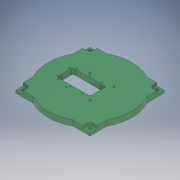
# Autodesk Inventor part: 000.202 - Крышка
Saved by Autodesk Inventor 2019 (Build 230136000, 136)
## iProperties
Created: 2020-03-17
Part Number: 000.202 - Крышка
Material: Пластик АБС
Document SubType Name: Modeling
Designer: Петров Иван
Density: 1.06 g/cm^3
Appearance: Гладкий — темный цвет морской волны
Author: Петров Иван
Autodesk Inventor part; units mm, degrees
ref_plane "YZ Plane" through (0, 0, 0) normal (1, 0, 0) x (0, 1, 0)
ref_plane "XZ Plane" through (0, 0, 0) normal (0, 1, 0) x (-1, 0, 0)
ref_plane "XY Plane" through (0, 0, 0) normal (0, 0, 1) x (1, 0, 0)
sketch "Эскиз1" plane through (0, 0, 0) normal (0, 0, 1) x (1, 0, 0)
  circle A0 centre (59.533, -59.533) radius 3 projected
  circle A1 centre (-59.533, -59.533) radius 3 projected
  circle A2 centre (-59.533, 59.533) radius 3 projected
  circle A3 centre (59.533, 59.533) radius 3 projected
  circle A4 centre (0, 0) radius 65 projected
  arc A5 (35.5618, 66.033) -> (-35.5618, 66.033) centre (0, 0) ccw projected
  line L0 (-35.5618, 66.033) -> (-66.033, 66.033) projected
  line L1 (-66.033, 66.033) -> (-66.033, 35.5618) projected
  arc A6 (-66.033, 35.5618) -> (-66.033, -35.5618) centre (0, 0) ccw projected
  line L2 (-66.033, -35.5618) -> (-66.033, -66.033) projected
  line L3 (-66.033, -66.033) -> (-35.5618, -66.033) projected
  arc A7 (-35.5618, -66.033) -> (35.5618, -66.033) centre (0, 0) ccw projected
  line L4 (35.5618, -66.033) -> (66.033, -66.033) projected
  line L5 (66.033, -66.033) -> (66.033, -35.5618) projected
  arc A8 (66.033, -35.5618) -> (66.033, 35.5618) centre (0, 0) ccw projected
  line L6 (66.033, 35.5618) -> (66.033, 66.033) projected
  line L7 (66.033, 66.033) -> (35.5618, 66.033) projected
  point P0 (0, 0)
extrude "Выдавливание1" add sketch "Эскиз1" along normal blind 10 contours A4 | L7 L6 A8 L5 L4 A7 L3 L2 A6 L1 L0 A5
sketch "Эскиз8" plane through (0, 0, 0) normal (0, 0, -1) x (-1, 0, 0)
  arc A0 (-18, 26.5) -> (-26.5, 18) centre (-18, 18) ccw
  line L0 (-26.5, -18) -> (-26.5, 18)
  arc A1 (-26.5, -18) -> (-18, -26.5) centre (-18, -18) ccw
  line L1 (18, -26.5) -> (-18, -26.5)
  arc A2 (18, -26.5) -> (26.5, -18) centre (18, -18) ccw
  line L2 (26.5, 18) -> (26.5, -18)
  arc A3 (26.5, 18) -> (18, 26.5) centre (18, 18) ccw
  line L3 (-18, 26.5) -> (18, 26.5)
  circle A4 centre (-21.2132, 21.2132) radius 1.5
  circle A5 centre (-21.2132, -21.2132) radius 1.5
  circle A6 centre (21.2132, -21.2132) radius 1.5
  circle A7 centre (21.2132, 21.2132) radius 1.5
  circle A8 centre (0, 0) radius 22
  constraints: 9 centre point, 8 end point, 8 point on circle
extrude "Выдавливание6" cut sketch "Эскиз8" against normal blind 10 contours A4 | A5 | A6 | A7
sketch "Эскиз9" plane through (0, 0, 0) normal (0, 0, -1) x (-1, 0, 0)
  line L0 (20.1, -44.6) -> (20.1, 8.5)
  line L1 (20.1, 8.5) -> (15, 14.5)
  line L2 (11.5, 14.5) -> (15, 14.5)
  line L3 (11.5, 14.5) -> (-11.5, 14.5)
  line L4 (-15, 14.5) -> (-11.5, 14.5)
  line L5 (-15, 14.5) -> (-20.1, 8.5)
  line L6 (-20.1, 8.5) -> (-20.1, -44.6)
  line L7 (-20.1, -44.6) -> (-15, -50.6)
  line L8 (-15, -50.6) -> (15, -50.6)
  line L9 (15, -50.6) -> (20.1, -44.6)
  circle A0 centre (11, -47.8) radius 1.025
  circle A1 centre (-11, -47.8) radius 1.025
  circle A2 centre (-17.3, -40) radius 1.025
  circle A3 centre (17.3, -40) radius 1.025
  circle A4 centre (17.3, -18) radius 1.025
  circle A5 centre (17.3, 4) radius 1.025
  circle A6 centre (-17.3, 4) radius 1.025
  circle A7 centre (0, 0) radius 1.55
  circle A8 centre (0, 0) radius 14
  line L10 (-14.5, 11.5) -> (-14.5, -42)
  arc A9 (-11.5, 14.5) -> (-14.5, 11.5) centre (-11.5, 11.5) ccw
  arc A10 (-14.5, -42) -> (-11.5, -45) centre (-11.5, -42) ccw
  line L11 (-20.1, 8.5) -> (-20.1, -44.6)
  arc A11 (14.5, 11.5) -> (11.5, 14.5) centre (11.5, 11.5) ccw
  line L12 (14.5, -42) -> (14.5, 11.5)
  arc A12 (11.5, -45) -> (14.5, -42) centre (11.5, -42) ccw
  line L13 (-11.5, -45) -> (11.5, -45)
  circle A13 centre (-17.3, -18) radius 1.025
  constraints: 28 end point, 14 centre point, 8 point on circle
extrude "Выдавливание7" cut sketch "Эскиз9" against normal blind 20.75 contours A11 L12 A12 L13 A10 L10 A9 L3 | A0 | A1 | A2 | A3 | A4 | A5 | A6 | A7 | A8 | A13
sketch "Эскиз10" plane through (0, 0, 0) normal (0, 0, -1) x (-1, 0, 0)
  circle A0 centre (59.533, -59.533) radius 3 projected
  circle A1 centre (59.533, -59.533) radius 6.5
  line L0 (66.033, -66.033) -> (35.5618, -66.033) projected
  line L1 (66.033, -35.5618) -> (66.033, -66.033) projected
  line L2 (59.533, -53.033) -> (66.033, -53.033)
  line L3 (66.033, -53.033) -> (66.033, -66.033)
  line L4 (66.033, -66.033) -> (53.033, -66.033)
  line L5 (53.033, -66.033) -> (53.033, -59.533)
  point P0 (0, 0)
  constraints: 8 end point, 2 parallel, 2 point on circle, 1 centre point, 1 coincident, 1 horizontal, 1 perpendicular, 1 tangent
extrude "Выдавливание8" cut sketch "Эскиз10" against normal blind 5
pattern_circular "Круговой массив1" count 4 over 360 about axis through (0, 0, 0) along (0, 0, 1) of "Выдавливание8"
